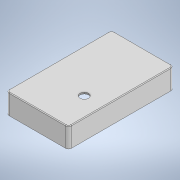
# Autodesk Inventor part: wanne
Saved by Autodesk Inventor 2022 (Build 260153000, 153)
## iProperties
Created: 2022-04-04
Part Number: wanne
Material: Generisch
Document SubType Name: Modeling
Designer: ga76xid
Density: 1 g/cm^3
Appearance: Vorgabe
Author: ga76xid
Autodesk Inventor part; units mm, degrees
ref_plane "YZ Plane" through (0, 0, 0) normal (1, 0, 0) x (0, 1, 0)
ref_plane "XZ Plane" through (0, 0, 0) normal (0, 1, 0) x (-1, 0, 0)
ref_plane "XY Plane" through (0, 0, 0) normal (0, 0, 1) x (1, 0, 0)
sketch "Skizze1" plane through (0, 0, 0) normal (0, 1, 0) x (-1, 0, 0)
  line L0 (1, 0) -> (40, 0)
  line L1 (41, 1) -> (41, 70)
  line L2 (40, 71) -> (1, 71)
  line L3 (0, 70) -> (0, 1)
  line L4 (42.2, 70.2) -> (42.2, 0.8)
  line L5 (40.2, -1.2) -> (0.8, -1.2)
  line L6 (-1.2, 0.8) -> (-1.2, 70.2)
  line L7 (0.8, 72.2) -> (40.2, 72.2)
  arc A0 (42.2, 70.2) -> (40.2, 72.2) centre (40.2, 70.2) ccw
  arc A1 (40.2, -1.2) -> (42.2, 0.8) centre (40.2, 0.8) ccw
  arc A2 (-1.2, 0.8) -> (0.8, -1.2) centre (0.8, 0.8) ccw
  arc A3 (0.8, 72.2) -> (-1.2, 70.2) centre (0.8, 70.2) ccw
  arc A4 (41, 70) -> (40, 71) centre (40, 70) ccw
  arc A5 (40, 0) -> (41, 1) centre (40, 1) ccw
  arc A6 (0, 1) -> (1, 0) centre (1, 1) ccw
  arc A7 (1, 71) -> (0, 70) centre (1, 70) ccw
  point P0 (0, 0)
  point P1 (41, 71)
  point P2 (41, 0)
  point P3 (0, 71)
  dimension "d0" = 41
  dimension "d1" = 71
  dimension "d2" = 1.2
  dimension "d3" = 2
  dimension "d4" = 1
  constraints: 16 end point, 16 point on circle, 16 tangent, 8 centre point, 8 point on line, 6 equal radius, 4 parallel, 2 perpendicular, 1 horizontal, 3 other
  measures "d0" distance of point (0, 71) point (41, 71)
  measures "d1" distance of point (41, 71) point (41, 0)
  measures "d2" distance between parallel lines of L1 L4
  measures "d3" radius of A0
  measures "d4" radius of A4
extrude "Extrusion1" add sketch "Skizze1" along normal blind 13
sketch "Skizze2" plane through (0, 13, 0) normal (0, 1, 0) x (1, 0, 0)
  line L0 (1.2, -70.2) -> (1.2, -0.8) projected
  arc A0 (1.2, -0.8) -> (-0.8, 1.2) centre (-0.8, -0.8) ccw projected
  line L1 (-0.8, 1.2) -> (-40.2, 1.2) projected
  arc A1 (-40.2, 1.2) -> (-42.2, -0.8) centre (-40.2, -0.8) ccw projected
  line L2 (-42.2, -0.8) -> (-42.2, -70.2) projected
  arc A2 (-42.2, -70.2) -> (-40.2, -72.2) centre (-40.2, -70.2) ccw projected
  line L3 (-40.2, -72.2) -> (-0.8, -72.2) projected
  arc A3 (-0.8, -72.2) -> (1.2, -70.2) centre (-0.8, -70.2) ccw projected
  arc A4 (0, -1) -> (-1, 0) centre (-1, -1) ccw projected
  line L4 (0, -1) -> (0, -70) projected
  arc A5 (-1, -71) -> (0, -70) centre (-1, -70) ccw projected
  line L5 (-1, -71) -> (-40, -71) projected
  arc A6 (-41, -70) -> (-40, -71) centre (-40, -70) ccw projected
  line L6 (-41, -70) -> (-41, -1) projected
  arc A7 (-40, 0) -> (-41, -1) centre (-40, -1) ccw projected
  line L7 (-40, 0) -> (-1, 0) projected
  point P0 (0, 0)
extrude "Extrusion2" add sketch "Skizze2" along normal blind 1 contours A3 L3 A2 L2 A1 L1 A0 L0 | L4 A5 L5 A6 L6 A7 L7 A4
fillet "Rundung1" radius 0.5 8 edges at (0.6142, 14, -0.6142) (-20.5, 14, -1.2) (-41.6142, 14, -0.6142) (-42.2, 14, 35.5) (-41.6142, 14, 71.6142) (-20.5, 14, 72.2) (0.6142, 14, 71.6142) (1.2, 14, 35.5)
sketch "Skizze3" plane through (0, 14, 0) normal (0, 1, 0) x (1, 0, 0)
  circle A0 centre (-12, -48) radius 3
  line L0 (0, -1) -> (0, -70) projected
  line L1 (-40, 0) -> (-1, 0) projected
  point P0 (0, 0)
  dimension "d10" = 6
  dimension "d11" = 12
  dimension "d12" = 48
  constraints: 1 centre point
  measures "d10" diameter of A0
  measures "d11" distance from line of L0 A0.centre
  measures "d12" distance from line of L1 A0.centre
extrude "Extrusion3" cut sketch "Skizze3" against normal blind 1
sketch "Skizze4" plane through (-0.8, 0, -1.2) normal (0, 0, -1) x (-1, 0, 0)
  circle A0 centre (26.4, 6.5) radius 4.5
  line L0 (0, 0) -> (39.4, 0) projected
  line L1 (41.4, 0) -> (41.4, 13.5) projected
  circle A1 centre (36.4, 6) radius 1.5
  point P0 (-0.8, 0)
  dimension "d15" = 9
  dimension "d16" = 6.5
  dimension "d17" = 15
  dimension "d18" = 3
  dimension "d19" = 5
  constraints: 2 centre point
  measures "d15" diameter of A0
  measures "d16" distance from line of L0 A0.centre
  measures "d17" distance from line of L1 A0.centre
  measures "d18" diameter of A1
  measures "d19" distance from line of L1 A1.centre
extrude "Extrusion4" cut sketch "Skizze4" against normal blind 5
